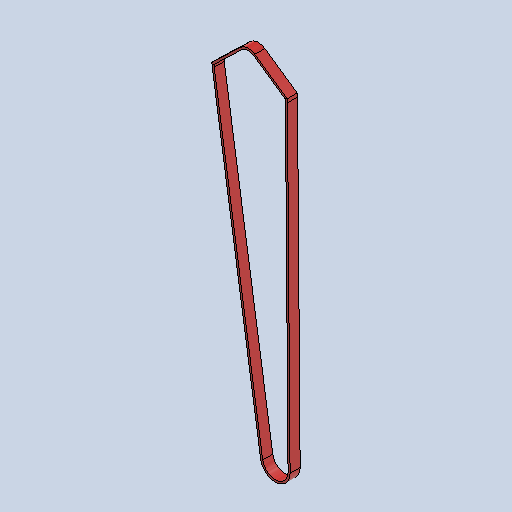
# Autodesk Inventor part: Compression bar band
Saved by Autodesk Inventor 2023.2 (Build 272271030, 271C)
## iProperties
Created: 2023-04-07
Part Number: Compression bar band
Material: Generic
Document SubType Name: Modeling
Designer: Main Account
Density: 1 g/cm^3
Appearance: Default
Author: Main Account
Autodesk Inventor part; units mm, degrees
ref_plane "YZ Plane" through (0, 0, 0) normal (1, 0, 0) x (0, 1, 0)
ref_plane "XZ Plane" through (0, 0, 0) normal (0, 1, 0) x (-1, 0, 0)
ref_plane "XY Plane" through (0, 0, 0) normal (0, 0, 1) x (1, 0, 0)
sketch "Sketch1" plane through (0, 0, 0) normal (0, 0, 1) x (1, 0, 0)
  circle A0 centre (-6, 6) radius 6.35 construction
  arc A1 (-12.2764, 5.0357) -> (0.3498, 6.0523) centre (-6, 6) ccw
  circle A2 centre (-19.4455, 172.9935) radius 4.7625 construction
  arc A3 (-16.7412, 176.9138) -> (-22.7422, 176.4306) centre (-19.4455, 172.9935) ccw
  line L0 (-36.4038, 162.0723) -> (-36.4975, 163.237) construction
  line L1 (-1.0522, 166.0908) -> (-0.9585, 164.9262) construction
  line L2 (-22.7422, 176.4306) -> (-36.4975, 163.237)
  line L3 (0.3498, 6.0523) -> (-0.9585, 164.9262)
  line L4 (-1.0522, 166.0908) -> (-0.9585, 164.9262)
  line L5 (-1.0522, 166.0908) -> (-16.7412, 176.9138)
  line L6 (-36.4975, 163.237) -> (-36.4038, 162.0723)
  line L7 (-36.4038, 162.0723) -> (-12.2764, 5.0357)
  line L8 (0.0412, 164.9705) -> (1.3498, 6.0605)
  arc A4 (-13.2648, 4.8838) -> (1.3498, 6.0605) centre (-6, 6) ccw
  line L9 (-13.2648, 4.8838) -> (-37.3976, 161.9561)
  line L10 (-37.3976, 161.9561) -> (-37.5324, 163.63)
  line L11 (-37.5324, 163.63) -> (-23.4345, 177.1523)
  arc A5 (-16.1734, 177.7369) -> (-23.4345, 177.1523) centre (-19.4455, 172.9935) ccw
  line L12 (-16.1734, 177.7369) -> (-0.0936, 166.6444)
  line L13 (-0.0936, 166.6444) -> (0.0412, 164.9705)
  point P0 (0, 0)
  dimension "d7" = 1
  constraints: 24 end point, 8 point on circle, 4 centre point, 4 tangent, 2 coincident, 2 concentric, 1 collinear, 7 other
  measures "d7" distance between parallel lines of L3 L8
extrude "Extrusion1" add sketch "Sketch1" along normal blind 5
body "Solid1"
